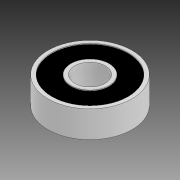
# Autodesk Inventor part: 608 bearing
Saved by Autodesk Inventor 2020 (Build 240168000, 168)
## iProperties
Created: 2021-03-19
Part Number: 608 bearing
Material: Generic
Document SubType Name: Modeling
Designer: DDeGo
Density: 1 g/cm^3
Appearance: Default
Author: DDeGo
Autodesk Inventor part; units mm, degrees
ref_plane "YZ Plane" through (0, 0, 0) normal (1, 0, 0) x (0, 1, 0)
ref_plane "XZ Plane" through (0, 0, 0) normal (0, 1, 0) x (-1, 0, 0)
ref_plane "XY Plane" through (0, 0, 0) normal (0, 0, 1) x (1, 0, 0)
sketch "Sketch1" plane through (0, 0, 0) normal (1, 0, 0) x (0, 1, 0)
  line L0 (0, 0) -> (7, 0) construction
  line L1 (7, 0) -> (7, -4) construction
  line L2 (7, -4) -> (0, -4)
  line L3 (0, -4) -> (0, 0) construction
  line L4 (7, -11) -> (0, -11)
  line L5 (7, -5) -> (6.8, -5)
  line L6 (6.8, -5) -> (6.8, -10)
  line L7 (6.8, -10) -> (7, -10)
  line L8 (0, -5) -> (0.2, -5)
  line L9 (0.2, -5) -> (0.2, -10)
  line L10 (0.2, -10) -> (0, -10)
  line L11 (7, -4) -> (7, -5)
  line L12 (7, -10) -> (7, -11)
  line L13 (0, -11) -> (0, -10)
  line L14 (0, -5) -> (0, -4)
  dimension "d0" = 4
  dimension "d2" = 7
  dimension "d5" = 11
  dimension "d6" = 0.2
  dimension "d7" = 1
  constraints: 30 end point, 7 perpendicular, 4 collinear, 4 point on line, 3 horizontal, 3 vertical
  measures "d0" distance between parallel lines of L0 L2
  measures "d2" distance of L0.start L0.end
  measures "d5" distance between parallel lines of L0 L4
  measures "d6" distance of L8.start L8.end
  measures "d7" distance of L8.start L2.end
revolve "Revolution1" add sketch "Sketch1" angle 360 about axis through (0, 0, 0) along (0, 1, 0)
body "Solid1"
